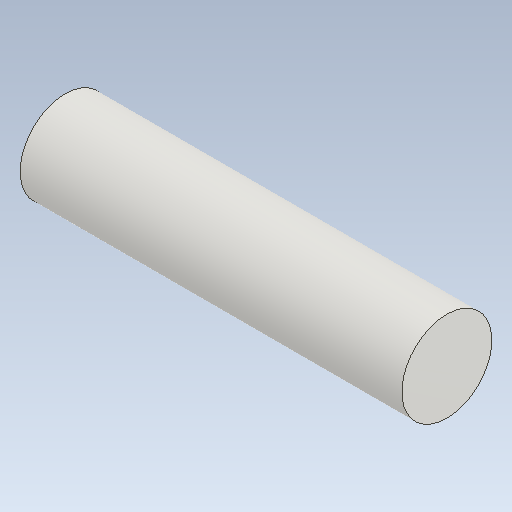
# Autodesk Inventor part: Shaft
Saved by Autodesk Inventor 2021 (Build 250183000, 183)
## iProperties
Created: 2021-03-10
Part Number: Shaft
Material: Steel
Document SubType Name: Modeling
Designer: M3rob
Density: 1 g/cm^3
Appearance: Steel
CustomPartVersion: 1
Author: M3rob
Length: 4.239 in
Autodesk Inventor part; units mm, degrees
ref_plane "Start Plane" through (0, 0, 0) normal (1, 0, 0) x (0, 1, 0)
ref_plane "XZ Plane" through (0, 0, 0) normal (0, 1, 0) x (-1, 0, 0)
ref_plane "XY Plane" through (0, 0, 0) normal (0, 0, 1) x (1, 0, 0)
sketch "Main Sketch" plane through (0, 0, 0) normal (0, 0, 1) x (1, 0, 0)
  line L0 (0, 0) -> (107.6726, 0)
  line L1 (0, 0) -> (0, 12.7)
  line L2 (0, 12.7) -> (100.1502, 12.7)
  line L3 (107.6726, 12.7) -> (107.6726, 0)
  line L4 (100.1502, 12.7) -> (107.6726, 12.7)
  dimension "d3" = 25.4
  dimension "d4" = 25.4
  constraints: 10 end point, 4 horizontal, 2 vertical
  measures "d3" diameter of L2 L0
  measures "d4" diameter of L4 L0
revolve "Revolution1" add sketch "Main Sketch" angle 360 about axis through (0, 0, 0) along (1, 0, 0)
equation "\"Length\" = 107.6706"
body "Solid1"
